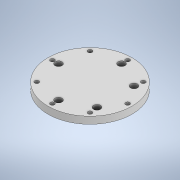
# Autodesk Inventor part: mountingPlate
Saved by Autodesk Inventor 2021 (Build 250183000, 183)
## iProperties
Created: 2021-01-06
Part Number: mountingPlate
Material: Generic
Document SubType Name: Modeling
Designer: awitc
Density: 1 g/cm^3
Appearance: Default
Author: awitc
Autodesk Inventor part; units mm, degrees
ref_plane "YZ Plane" through (0, 0, 0) normal (1, 0, 0) x (0, 1, 0)
ref_plane "XZ Plane" through (0, 0, 0) normal (0, 1, 0) x (-1, 0, 0)
ref_plane "XY Plane" through (0, 0, 0) normal (0, 0, 1) x (1, 0, 0)
sketch "Sketch1" plane through (0, 0, 0) normal (0, 1, 0) x (-1, 0, 0)
  circle A0 centre (26.875, 0) radius 1.5
  circle A1 centre (0, -26.875) radius 1.5
  circle A2 centre (-26.875, 0) radius 1.5
  circle A3 centre (0, 26.875) radius 1.5
  circle A4 centre (19.0035, 19.0035) radius 1.5
  circle A5 centre (19.0035, -19.0035) radius 1.5
  circle A6 centre (-19.0035, -19.0035) radius 1.5
  circle A7 centre (-19.0035, 19.0035) radius 1.5
  circle A8 centre (0, 0) radius 28.75
  circle A9 centre (0, 0) radius 30
  point P0 (-23.5374, 22.0452)
  dimension "d9" = 3
  dimension "d10" = 3
  dimension "d11" = 3
  dimension "d12" = 3
  dimension "d13" = 3
  dimension "d14" = 3
  dimension "d15" = 3
  dimension "d16" = 3
  dimension "d17" = 57.5
  dimension "d33" = 60
  constraints: 10 centre point, 1 coincident
  measures "d9" diameter of A0
  measures "d10" diameter of A1
  measures "d11" diameter of A2
  measures "d12" diameter of A3
  measures "d13" diameter of A4
  measures "d14" diameter of A5
  measures "d15" diameter of A6
  measures "d16" diameter of A7
  measures "d17" diameter of A8
  measures "d33" diameter of A9
extrude "Extrusion1" add sketch "Sketch1" along normal blind 5 contours A8 | A9
sketch "Sketch2" plane through (0, 5, 0) normal (0, 1, 0) x (1, 0, 0)
  circle A0 centre (0, 0) radius 25
  line L0 (22.1416, 4) -> (20.8701, 4)
  line L1 (22.1416, -4) -> (20.8701, -4)
  arc A1 (24.6779, 4) -> (-17.6137, 17.7414) centre (0, 0) ccw
  arc A2 (-17.6137, -17.7414) -> (24.6779, -4) centre (0, 0) ccw
  line L2 (24.6779, -4) -> (22.1416, -4)
  line L3 (24.6779, 4) -> (22.1416, 4)
  line L4 (-15.5618, -16.2506) -> (-14.5332, -15.5032)
  line L5 (-19.2354, -9.0311) -> (-15.1903, -6.0922)
  line L6 (-15.1903, -6.0922) -> (-10.4881, -12.5643)
  line L7 (-10.4881, -12.5643) -> (-14.5332, -15.5032)
  line L8 (-22.316, -11.2693) -> (-20.2641, -9.7784)
  line L9 (-17.6137, -17.7414) -> (-15.5618, -16.2506)
  line L10 (-20.2641, -9.7784) -> (-19.2354, -9.0311)
  circle A3 centre (0, 22.5) radius 1.5
  line L11 (-10.4881, 12.5643) -> (-15.1903, 6.0922)
  line L12 (-14.5332, 15.5032) -> (-10.4881, 12.5643)
  line L13 (-15.5618, 16.2506) -> (-14.5332, 15.5032)
  line L14 (-15.1903, 6.0922) -> (-19.2354, 9.0311)
  line L15 (-20.2641, 9.7784) -> (-19.2354, 9.0311)
  line L16 (-17.6137, 17.7414) -> (-15.5618, 16.2506)
  line L17 (-23.5374, 22.0452) -> (-13.679, 22.0452) construction
  line L18 (-22.316, 11.2693) -> (-20.2641, 9.7784)
  arc A4 (-22.316, 11.2693) -> (-22.316, -11.2693) centre (0, 0) ccw
  line L19 (15.8701, -4) -> (20.8701, -4)
  circle A5 centre (18.2029, -13.2252) radius 1.5
  circle A6 centre (0, -22.5) radius 1.5
  circle A7 centre (18.2029, 13.2252) radius 1.5
  line L20 (20.8701, 4) -> (15.8701, 4)
  line L21 (15.8701, 4) -> (15.8701, -4)
  arc A8 (-13.5023, -14.7543) -> (19.5959, -4) centre (0, 0) ccw
  arc A9 (19.5959, 4) -> (-13.5023, 14.7543) centre (0, 0) ccw
  arc A10 (-18.2046, 8.2821) -> (-18.2046, -8.2821) centre (0, 0) ccw
  circle A11 centre (-22.5, 0) radius 1.5
  circle A12 centre (0, 0) radius 20
  circle A13 centre (-22.5, 0) radius 2.5
  circle A14 centre (0, -22.5) radius 2.5
  circle A15 centre (18.2029, -13.2252) radius 2.5
  circle A16 centre (18.2029, 13.2252) radius 2.5
  circle A17 centre (0, 22.5) radius 2.5
  point P0 (-28.2397, -15.5731)
  point P1 (-23.5374, -22.0452)
  dimension "d20" = 50
  dimension "d21" = 36
  dimension "d22" = 5
  dimension "d23" = 5
  dimension "d24" = 3
  dimension "d25" = 3
  dimension "d26" = 3
  dimension "d27" = 3
  dimension "d28" = 3
  dimension "d29" = 5
  dimension "d30" = 5
  constraints: 44 end point, 18 centre point, 12 point on circle, 7 coincident, 6 point on line, 5 parallel, 4 perpendicular, 3 horizontal, 2 tangent
  measures "d20" diameter of A0
  measures "d21" angle of L16 L17
  measures "d22" distance of L19.end L19.start
  measures "d23" distance of L12.start L11.start
  measures "d24" diameter of A3
  measures "d25" diameter of A7
  measures "d26" diameter of A5
  measures "d27" diameter of A6
  measures "d28" diameter of A11
  measures "d29" diameter of A13
  measures "d30" diameter of A16
extrude "Extrusion2" cut sketch "Sketch2" against normal blind 3 contours A16 | A15 | A17 | A14 | A13 | A3 | A5 | A6 | A7 | A11
sketch "Sketch3" plane through (0, 0, 0) normal (0, -1, 0) x (1, 0, 0)
  circle A0 centre (0, 0) radius 20
  circle A1 centre (0, 0) radius 10
  circle A2 centre (0, 15.75) radius 2.5
  circle A3 centre (15.75, 0) radius 2.5
  line L0 (0, 0) -> (11.1369, 11.1369)
  line L1 (0, 0) -> (15.75, 0) construction
  circle A4 centre (11.1369, 11.1369) radius 2.5
  circle A5 centre (11.1369, -11.1369) radius 2.5
  circle A6 centre (-11.1369, -11.1369) radius 2.5
  circle A7 centre (-11.1369, 11.1369) radius 2.5
  circle A8 centre (-15.75, 0) radius 2.5
  circle A9 centre (0, -15.75) radius 2.5
  dimension "d34" = 40
  dimension "d35" = 20
  dimension "d37" = 5
  dimension "d38" = 5
  dimension "d39" = 45
  dimension "d40" = 5
  dimension "d41" = 5
  dimension "d42" = 5
  dimension "d43" = 5
  dimension "d44" = 5
  dimension "d45" = 5
  constraints: 10 centre point, 4 coincident, 4 end point, 1 equal length, 1 horizontal
  measures "d34" diameter of A0
  measures "d35" diameter of A1
  measures "d37" diameter of A2
  measures "d38" diameter of A3
  measures "d39" angle of L1 L0
  measures "d40" diameter of A4
  measures "d41" diameter of A5
  measures "d42" diameter of A6
  measures "d43" diameter of A7
  measures "d44" diameter of A8
  measures "d45" diameter of A9
extrude "Extrusion3" add sketch "Sketch3" along normal blind 5
body "Solid1"
